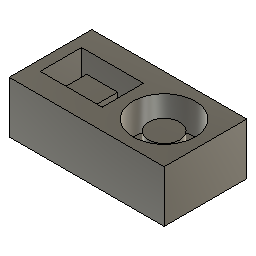
Probe testing (Autodesk Fusion 360 design; units mm, degrees)
Autodesk Fusion 360 part; units mm, degrees
box "BoxPrimitive1" add length 40 width 75 height 25 placed x (0, 1, 0) y (-1, 0, 0) z (0, 0, 1) at (75, 0, 0)
sketch "Sketch2" plane through (0, 0, 25) normal (0, 0, 1) x (-1, 0, 0)
  line L0 (-5, -30) -> (-35, -30)
  line L1 (-35, -30) -> (-35, -10)
  line L2 (-35, -10) -> (-5, -10)
  line L3 (-5, -10) -> (-5, -30)
  line L4 (-12.5, -25) -> (-27.5, -25)
  line L5 (-27.5, -25) -> (-27.5, -15)
  line L6 (-27.5, -15) -> (-12.5, -15)
  line L7 (-12.5, -15) -> (-12.5, -25)
  circle A0 centre (-55, -20) radius 15
  circle A1 centre (-55, -20) radius 7.5
  line L8 (0, 0) -> (0, -40) construction
  line L9 (-75, -40) -> (-75, 0) construction
  line L10 (0, -20) -> (-75, -20) construction
  line L11 (-35, -20) -> (-12.5, -20) construction
  line L12 (-20, -25) -> (-20, -30) construction
  dimension "d6" = 30
  dimension "d7" = 15
  dimension "d8" = 20
  dimension "d9" = 20
  dimension "d10" = 10
  dimension "d11" = 30
  dimension "d12" = 15
  dimension "d13" = 20
  measures "d6" diameter of A0
  measures "d7" diameter of A1
  measures "d11" distance of L8.start
  measures "d12" distance of L8.start
  measures "d13" distance of L8 L12
extrude "Extrude1" cut sketch "Sketch2" against normal blind 15
extrude "Extrude2" cut 2 faces at (56.8894, 23.4929, 25) (22.5, 21.6667, 25) along direction (0, 0, -1) blind 5
